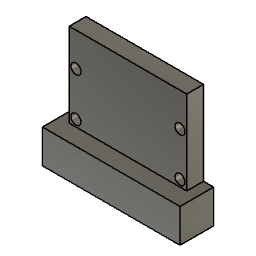
soporte cam v1 (Autodesk Fusion 360 design; units mm, degrees)
Autodesk Fusion 360 part; units mm, degrees
sketch "Sketch1" plane through (0, 0, 0) normal (0, 0, 1) x (1, 0, 0)
  line L0 (-50, 0) -> (-15, 0)
  line L1 (-15, 0) -> (-15, 10)
  line L2 (-15, 10) -> (-50, 10)
  line L3 (-50, 10) -> (-50, 0)
  dimension "d1" = 35
  dimension "d2" = 10
  constraint horizontal L0
  constraint vertical L1
  constraint horizontal L2
  constraint vertical L3
  measures "d1" distance of L0.start L0.end
  measures "d2" distance of L0.start L2.end
extrude "Extrude1" add sketch "Sketch1" along normal blind 10
sketch "Sketch2" plane through (0, 0, 10) normal (0, 0, 1) x (-1, 0, 0)
  line L0 (50, -10) -> (50, 0)
  line L1 (50, 0) -> (15, 0)
  line L2 (15, 0) -> (15, -10)
  line L3 (15, -10) -> (50, -10)
  line L4 (50, -10) -> (50, -5)
  line L5 (15, -5) -> (15, -10)
  line L6 (15, -5) -> (20, -5)
  line L7 (20, -5) -> (50, -5)
  line L8 (50, -10) -> (15, -10)
  constraint coincident L0.start L3.end
  constraint midpoint L0 L4.end
  constraint midpoint L2 L5.start
  constraint coincident L2.end L3.start
  constraint perpendicular L2 L6
  constraint perpendicular L0 L7
extrude "Extrude2" add sketch "Sketch2" along normal blind 25 contours L0 L2 L3 L4 L5 L6 L7 L8
sketch "Sketch3" plane through (0, 5, 0) normal (0, -1, 0) x (1, 0, 0)
  line L0 (-50, 10) -> (-15, 10)
  line L1 (-15, 10) -> (-15, 35)
  line L2 (-15, 35) -> (-50, 35)
  line L3 (-50, 35) -> (-50, 10)
  line L4 (-15, 10) -> (-17, 10)
  line L5 (-17, 10) -> (-17, 12)
  circle A0 centre (-17, 12) radius 1.5
  line L6 (-50, 10) -> (-48, 10)
  circle A1 centre (-48, 12) radius 1.5
  dimension "d7" = 2
  dimension "d8" = 2
  dimension "d9" = 3
  dimension "d10" = 2
  dimension "d11" = 3
  constraint coincident L0.end L1.start
  constraint horizontal L4
  constraint perpendicular L4 L5
  constraint coincident L5.end A0.centre
  constraint coincident L0.start L3.end
  constraint perpendicular L3 L6
  measures "d7" distance of L0.end L4.end
  measures "d8" distance of L4.end L5.end
  measures "d9" diameter of A0
  measures "d10" distance of L0.start L6.end
  measures "d11" diameter of A1
extrude "Extrude3" cut sketch "Sketch3" against normal blind 15 contours A0 | A1
sketch "Sketch4" plane through (0, 5, 0) normal (0, -1, 0) x (1, 0, 0)
  circle A0 centre (-17, 12) radius 1.5
  circle A1 centre (-48, 12) radius 1.5
  line L0 (-50, 10) -> (-15, 10)
  line L1 (-15, 10) -> (-15, 35)
  line L2 (-15, 35) -> (-50, 35)
  line L3 (-50, 35) -> (-50, 10)
  line L4 (-17, 10) -> (-17, 25)
  line L5 (-48, 10) -> (-48, 25)
  circle A2 centre (-48, 25) radius 1.5
  circle A3 centre (-17, 25) radius 1.5
  dimension "d14" = 15
  dimension "d15" = 15
  dimension "d16" = 3
  dimension "d17" = 3
  constraint coincident L0 L4.start
  constraint perpendicular L0 L4
  constraint coincident L0 L5.start
  constraint perpendicular L0 L5
  constraint coincident L5.end A2.centre
  constraint coincident L4.end A3.centre
  measures "d14" distance of L4.start L4.end
  measures "d15" distance of L5.start L5.end
  measures "d16" diameter of A2
  measures "d17" diameter of A3
extrude "Extrude4" cut sketch "Sketch4" against normal blind 24 contours A2 | A3
sketch "Sketch5" plane through (0, 0, 0) normal (0, 0, -1) x (1, 0, 0)
  line L0 (-50, 0) -> (-50, -10)
  line L1 (-50, -10) -> (-15, -10)
  line L2 (-15, -10) -> (-15, 0)
  line L3 (-15, 0) -> (-50, 0)
sketch "Sketch6" plane through (-50, 0, 0) normal (-1, 0, 0) x (0, -1, 0)
  line L0 (-10, 0) -> (0, 0)
  line L1 (0, 0) -> (0, 10)
  line L2 (0, 10) -> (-5, 10)
  line L3 (-5, 10) -> (-5, 35)
  line L4 (-5, 35) -> (-10, 35)
  line L5 (-10, 35) -> (-10, 0)
  line L6 (0, 10) -> (-10, 10)
  line L7 (-10, 10) -> (-10, 0)
  line L8 (-10, 0) -> (0, 0)
  line L9 (0, 0) -> (0, 10)
  constraint horizontal L6
  constraint vertical L7
  constraint horizontal L8
  constraint vertical L9
  constraint coincident L0.start L5.end
  constraint coincident L1.end L2.start
extrude "Extrude5" add sketch "Sketch6" along normal blind 3 contours L0 L1 L2 L5 L6 L7 L8 L9
sketch "Sketch7" plane through (-15, 0, 0) normal (1, 0, 0) x (0, 1, 0)
  line L0 (0, 0) -> (10, 0)
  line L1 (10, 0) -> (10, 35)
  line L2 (10, 35) -> (5, 35)
  line L3 (5, 35) -> (5, 10)
  line L4 (5, 10) -> (0, 10)
  line L5 (0, 10) -> (0, 0)
  line L6 (0, 10) -> (10, 10)
  line L7 (10, 10) -> (10, 0)
  line L8 (10, 0) -> (0, 0)
  line L9 (0, 0) -> (0, 10)
  constraint horizontal L6
  constraint vertical L7
  constraint horizontal L8
  constraint vertical L9
  constraint coincident L0.end L1.start
  constraint coincident L4.end L5.start
extrude "Extrude6" add sketch "Sketch7" along normal blind 3 contours L0 L1 L4 L5 L6 L7 L8 L9
sketch "Sketch8" plane through (0, 0, 0) normal (0, 0, -1) x (1, 0, 0)
sketch "Sketch9" plane through (0, 0, 0) normal (0, 0, -1) x (1, 0, 0)
  line L0 (-53, -10) -> (-52, -10)
  line L1 (-52, -10) -> (-32, -10)
  line L2 (-32, -10) -> (-32, -5)
  line L3 (-32, -5) -> (-15, -5)
  line L4 (-32, -5) -> (-49, -5)
  line L5 (-49, -5) -> (-49, -1)
  line L6 (-49, -5) -> (-49, -9)
  line L7 (-49, -1) -> (-15, -1)
  line L8 (-15, -1) -> (-15, -9)
  line L9 (-15, -9) -> (-49, -9)
  dimension "d24" = 20
  dimension "d25" = 17
  dimension "d26" = 17
  dimension "d27" = 4
  dimension "d28" = 4
  constraint horizontal L0
  constraint parallel L0 L1
  constraint perpendicular L1 L2
  constraint perpendicular L2 L3
  constraint perpendicular L2 L4
  constraint perpendicular L4 L5
  constraint perpendicular L4 L6
  constraint perpendicular L5 L7
  constraint perpendicular L1 L8
  constraint perpendicular L6 L9
  measures "d24" distance of L0.end L1.end
  measures "d25" distance of L2.end L3.end
  measures "d26" distance of L2.end L4.end
  measures "d27" distance of L4.end L5.end
  measures "d28" distance of L4.end L6.end
extrude "Extrude7" cut sketch "Sketch9" against normal blind 5
